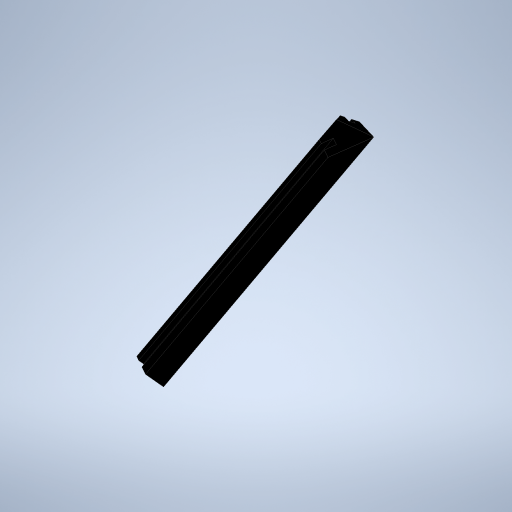
# Autodesk Inventor part: Perfil_V2
Saved by Autodesk Inventor 2024 (Build 280153000, 153)
## iProperties
Created: 2023-07-27
Part Number: Perfil_V2
Material: Genérico
Document SubType Name: Modeling
Designer: sergi
Density: 1 g/cm^3
Appearance: Valor por defecto
Author: sergi
Autodesk Inventor part; units mm, degrees
sketch "Boceto1" plane through (0, 0, 0) normal (0, 1, 0) x (-1, 0, 0)
  line L0 (65, 89.4648) -> (105.1722, -34.1725)
  line L1 (105.1722, -34.1725) -> (0, -110.5846)
  line L2 (0, -110.5846) -> (-105.1722, -34.1725)
  line L3 (-105.1722, -34.1725) -> (-65, 89.4648)
  line L4 (-65, 89.4648) -> (65, 89.4648)
  line L5 (0, 0) -> (178.9296, 0) construction
  line L6 (178.9296, 0) -> (178.9296, 178.9296) construction
  line L7 (178.9296, 178.9296) -> (0, 178.9296) construction
  line L8 (0, 178.9296) -> (0, 0) construction
  line L9 (178.9296, 178.9296) -> (0, 89.4648)
  dimension "d1" = 289.5143
  dimension "d2" = 26.565
  dimension "d108" = 130
  constraints: 20 end point, 2 horizontal, 2 midpoint, 2 parallel, 2 perpendicular, 1 coincident, 11 other
  measures "d1" distance from line of L1.end L7
  measures "d2" angle of L4 L9
  measures "d108" distance of L3.end L0.start
extrude "Extrusión1" add sketch "Boceto1" along normal blind 289.5143 draft 26.565
sketch "Boceto2" plane through (0, 289.5143, 0) normal (0, 1, 0) x (1, 0, 0)
  line L0 (0, -80.8118) -> (-76.8566, -24.9722)
  line L1 (-76.8566, -24.9722) -> (-47.5, 65.3781)
  line L2 (-47.5, 65.3781) -> (47.5, 65.3781)
  line L3 (47.5, 65.3781) -> (76.8566, -24.9722)
  line L4 (76.8566, -24.9722) -> (0, -80.8118)
  point P0 (0, 0)
  point P1 (0, 0)
  dimension "L" = 95
  constraints: 10 end point, 1 coincident, 1 horizontal, 11 other
  measures "L" distance of L1.end L2.end
extrude "Extrusión2" cut sketch "Boceto2" against normal blind 289.5143 draft 26.565 keep common part
sketch "Boceto3" plane through (65, 0, 89.4648) normal (0.8506508, -0.4472136, 0.2763932) x (0.309017, 0, -0.9510565)
  line L0 (65, 170.2767) -> (162.346, 99.5507) projected
  line L1 (-32.346, 99.5507) -> (65, 170.2767) projected
  line L2 (0, 0) -> (-32.346, 99.5507) projected
  line L3 (0, 0) -> (130, 0) projected
  line L4 (130, 0) -> (162.346, 99.5507) projected
  line L5 (151.1781, 95.922) -> (65, 158.534)
  line L6 (65, 158.534) -> (-21.1781, 95.922)
  line L7 (-21.1781, 95.922) -> (6.9022, 9.5)
  line L8 (6.9022, 9.5) -> (123.0978, 9.5)
  line L9 (123.0978, 9.5) -> (151.1781, 95.922)
  point P0 (65, -40.0099)
  dimension "D" = 9.5
  constraints: 10 end point, 4 other
  measures "D" distance between parallel lines of L4 L9
extrude "Extrusión3" cut sketch "Boceto3" against normal blind 189.5143 contours L9 L8 L7 L6 L5
sketch "Boceto4" plane through (105.1722, 0, -34.1725) normal (0.5257311, -0.4472136, -0.7236068) x (-0.809017, 0, -0.5877853)
  line L0 (65, 170.2767) -> (162.346, 99.5507) projected
  line L1 (-32.346, 99.5507) -> (65, 170.2767) projected
  line L2 (0, 0) -> (-32.346, 99.5507) projected
  line L3 (0, 0) -> (130, 0) projected
  line L4 (130, 0) -> (162.346, 99.5507) projected
  line L5 (123.0978, 9.5) -> (6.9022, 9.5)
  line L6 (6.9022, 9.5) -> (-21.1781, 95.922)
  line L7 (-21.1781, 95.922) -> (65, 158.534)
  line L8 (65, 158.534) -> (151.1781, 95.922)
  line L9 (151.1781, 95.922) -> (123.0978, 9.5)
  point P0 (65, -40.0099)
  dimension "d14" = 9.5
  constraints: 10 end point, 4 other
  measures "d14" distance between parallel lines of L3 L5
extrude "Extrusión4" cut sketch "Boceto4" against normal blind 189.5143 contours L5 L6 L7 L8 L9
sketch "Boceto5" plane through (0, 0, 0) normal (0, -1, 0) x (1, 0, 0)
  line L0 (105.1722, -34.1725) -> (0, -110.5846) projected
  line L1 (65, 89.4648) -> (105.1722, -34.1725) projected
  line L2 (-65, 89.4648) -> (65, 89.4648) projected
  line L3 (-105.1722, -34.1725) -> (-65, 89.4648) projected
  line L4 (0, -110.5846) -> (-105.1722, -34.1725) projected
  line L5 (58.0978, 79.9648) -> (94.0043, -30.5438)
  line L6 (94.0043, -30.5438) -> (0, -98.842)
  line L7 (0, -98.842) -> (-94.0043, -30.5438)
  line L8 (-94.0043, -30.5438) -> (-58.0978, 79.9648)
  line L9 (-58.0978, 79.9648) -> (58.0978, 79.9648)
  point P0 (0, 0)
  dimension "d17" = 9.5
  constraints: 10 end point, 4 other
  measures "d17" distance between parallel lines of L2 L9
extrude "Extrusión5" cut sketch "Boceto5" against normal blind 189.5143 contours L5 L6 L7 L8 L9
sketch "Boceto6" plane through (47.5, 289.5143, -65.3781) normal (0, 0.4472136, -0.8944272) x (-1, 0, 0)
  line L0 (47.5, -224.1361) -> (144.846, -153.4101) projected
  line L1 (95, 0) -> (144.846, -153.4101) projected
  line L2 (95, 0) -> (0, 0) projected
  line L3 (0, 0) -> (-49.846, -153.4101) projected
  line L4 (-49.846, -153.4101) -> (47.5, -224.1361) projected
  line L5 (133.6781, -149.7814) -> (47.5, -212.3935)
  line L6 (47.5, -212.3935) -> (-38.6781, -149.7814)
  line L7 (-38.6781, -149.7814) -> (6.9022, -9.5)
  line L8 (6.9022, -9.5) -> (88.0978, -9.5)
  line L9 (88.0978, -9.5) -> (133.6781, -149.7814)
  point P0 (47.5, -229.7114)
  dimension "d20" = 9.5
  constraints: 10 end point, 4 other
  measures "d20" distance between parallel lines of L0 L5
extrude "Extrusión6" cut sketch "Boceto6" against normal blind 189.5143 contours L5 L6 L7 L8 L9
sketch "Boceto7" plane through (0, 0, -110.5846) normal (-0.5257311, -0.4472136, -0.7236068) x (-0.809017, 0, 0.5877853)
  line L0 (65, 170.2767) -> (162.346, 99.5507) projected
  line L1 (-32.346, 99.5507) -> (65, 170.2767) projected
  line L2 (0, 0) -> (-32.346, 99.5507) projected
  line L3 (0, 0) -> (130, 0) projected
  line L4 (130, 0) -> (162.346, 99.5507) projected
  line L5 (151.1781, 95.922) -> (65, 158.534)
  line L6 (65, 158.534) -> (-21.1781, 95.922)
  line L7 (-21.1781, 95.922) -> (6.9022, 9.5)
  line L8 (6.9022, 9.5) -> (123.0978, 9.5)
  line L9 (123.0978, 9.5) -> (151.1781, 95.922)
  point P0 (65, -40.0099)
  dimension "d23" = 9.5
  constraints: 10 end point, 4 other
  measures "d23" distance between parallel lines of L4 L9
extrude "Extrusión7" cut sketch "Boceto7" against normal blind 189.5143 contours L9 L8 L7 L6 L5
sketch "Boceto8" plane through (76.8566, 289.5143, 24.9722) normal (0.8506508, 0.4472136, -0.2763932) x (-0.309017, 0, -0.9510565)
  line L0 (47.5, -224.1361) -> (144.846, -153.4101) projected
  line L1 (95, 0) -> (144.846, -153.4101) projected
  line L2 (95, 0) -> (0, 0) projected
  line L3 (0, 0) -> (-49.846, -153.4101) projected
  line L4 (-49.846, -153.4101) -> (47.5, -224.1361) projected
  line L5 (47.5, -212.3935) -> (133.6781, -149.7814)
  line L6 (133.6781, -149.7814) -> (88.0978, -9.5)
  line L7 (88.0978, -9.5) -> (6.9022, -9.5)
  line L8 (6.9022, -9.5) -> (-38.6781, -149.7814)
  line L9 (-38.6781, -149.7814) -> (47.5, -212.3935)
  point P0 (47.5, -229.7114)
  dimension "d26" = 9.5
  constraints: 10 end point, 4 other
  measures "d26" distance between parallel lines of L4 L9
extrude "Extrusión8" cut sketch "Boceto8" against normal blind 189.5143 contours L9 L8 L7 L6 L5
sketch "Boceto9" plane through (0, 289.5143, 0) normal (0, 1, 0) x (1, 0, 0)
  line L0 (78.7643, -17.095) -> (-82.4461, -69.4755) projected
  line L1 (-47.5, 65.3781) -> (47.5, 65.3781) projected
  line L2 (-76.8566, -24.9722) -> (-47.5, 65.3781) projected
  line L3 (0, -80.8118) -> (-76.8566, -24.9722) projected
  line L4 (76.8566, -24.9722) -> (0, -80.8118) projected
  line L5 (47.5, 65.3781) -> (76.8566, -24.9722) projected
  line L6 (0, -69.0692) -> (-65.6887, -21.3436)
  line L7 (-65.6887, -21.3436) -> (-40.5978, 55.8781)
  line L8 (-40.5978, 55.8781) -> (40.5978, 55.8781)
  line L9 (40.5978, 55.8781) -> (65.6887, -21.3436)
  line L10 (65.6887, -21.3436) -> (0, -69.0692)
  point P0 (0, 0)
  dimension "d29" = 9.5
  constraints: 10 end point, 4 other
  measures "d29" distance between parallel lines of L4 L10
extrude "Extrusión9" cut sketch "Boceto9" against normal blind 189.5143 contours L10 L6 L0 | L0 L6 L7 L8 L9
sketch "Boceto10" plane through (-47.5, 289.5143, -65.3781) normal (-0.8506508, 0.4472136, -0.2763932) x (-0.309017, 0, 0.9510565)
  line L0 (-49.846, -153.4101) -> (47.5, -224.1361) projected
  line L1 (47.5, -224.1361) -> (144.846, -153.4101) projected
  line L2 (95, 0) -> (144.846, -153.4101) projected
  line L3 (95, 0) -> (0, 0) projected
  line L4 (0, 0) -> (-49.846, -153.4101) projected
  line L5 (133.6781, -149.7814) -> (47.5, -212.3935)
  line L6 (47.5, -212.3935) -> (-38.6781, -149.7814)
  line L7 (-38.6781, -149.7814) -> (6.9022, -9.5)
  line L8 (6.9022, -9.5) -> (88.0978, -9.5)
  line L9 (88.0978, -9.5) -> (133.6781, -149.7814)
  point P0 (47.5, -229.7114)
  dimension "d32" = 9.5
  constraints: 10 end point, 4 other
  measures "d32" distance between parallel lines of L2 L9
extrude "Extrusión10" cut sketch "Boceto10" against normal blind 189.5143 contours L5 L6 L7 L8 L9
sketch "Boceto11" plane through (-105.1722, 0, -34.1725) normal (-0.8506508, -0.4472136, 0.2763932) x (0.309017, 0, 0.9510565)
  line L0 (93.5693, 85.4327) -> (113.4241, 91.884) projected
  line L1 (-32.346, 99.5507) -> (65, 170.2767) projected
  line L2 (0, 0) -> (-32.346, 99.5507) projected
  line L3 (0, 0) -> (130, 0) projected
  line L4 (130, 0) -> (162.346, 99.5507) projected
  line L5 (65, 170.2767) -> (162.346, 99.5507) projected
  line L6 (151.1781, 95.922) -> (123.0978, 9.5)
  line L7 (123.0978, 9.5) -> (6.9022, 9.5)
  line L8 (6.9022, 9.5) -> (-21.1781, 95.922)
  line L9 (-21.1781, 95.922) -> (65, 158.534)
  line L10 (65, 158.534) -> (151.1781, 95.922)
  point P0 (65, -40.0099)
  point P1 (48.882, 67.2803)
  point P2 (90.6407, 79.3954)
  point P3 (78.7461, 79.1633)
  dimension "d35" = 9.5
  constraints: 10 end point, 5 other
  measures "d35" distance between parallel lines of L4 L6
extrude "Extrusión11" cut sketch "Boceto11" against normal blind 189.5143 contours L6 L7 L8 L9 L10
sketch "Boceto12" plane through (-65, 0, 89.4648) normal (0, -0.4472136, 0.8944272) x (1, 0, 0)
  line L0 (6.9022, 9.5) -> (97.7716, 134.5711) projected
  line L1 (-32.346, 99.5507) -> (65, 170.2767) projected
  line L2 (0, 0) -> (-32.346, 99.5507) projected
  line L3 (0, 0) -> (130, 0) projected
  line L4 (130, 0) -> (162.346, 99.5507) projected
  line L5 (65, 170.2767) -> (162.346, 99.5507) projected
  line L6 (151.1781, 95.922) -> (123.0978, 9.5)
  line L7 (123.0978, 9.5) -> (6.9022, 9.5)
  line L8 (6.9022, 9.5) -> (-21.1781, 95.922)
  line L9 (-21.1781, 95.922) -> (65, 158.534)
  line L10 (65, 158.534) -> (151.1781, 95.922)
  point P0 (65, -40.0099)
  point P1 (52.5, 72.2601)
  point P2 (45.5555, 62.7017)
  dimension "d38" = 9.5
  constraints: 10 end point, 4 other
  measures "d38" distance between parallel lines of L5 L10
extrude "Extrusión12" cut sketch "Boceto12" against normal blind 189.5143 contours L6 L7 L8 L9 L10
sketch "Boceto13" plane through (0, 289.5143, 80.8118) normal (0.5257311, 0.4472136, 0.7236068) x (0.809017, 0, -0.5877853)
  line L0 (-49.846, -153.4101) -> (47.5, -224.1361) projected
  line L1 (47.5, -224.1361) -> (144.846, -153.4101) projected
  line L2 (95, 0) -> (144.846, -153.4101) projected
  line L3 (95, 0) -> (0, 0) projected
  line L4 (0, 0) -> (-49.846, -153.4101) projected
  line L5 (47.5, -212.3935) -> (-38.6781, -149.7814)
  line L6 (-38.6781, -149.7814) -> (6.9022, -9.5)
  line L7 (6.9022, -9.5) -> (88.0978, -9.5)
  line L8 (88.0978, -9.5) -> (133.6781, -149.7814)
  line L9 (133.6781, -149.7814) -> (47.5, -212.3935)
  point P0 (47.5, -229.7114)
  dimension "d41" = 9.5
  constraints: 10 end point, 4 other
  measures "d41" distance between parallel lines of L0 L5
extrude "Extrusión13" cut sketch "Boceto13" against normal blind 189.5143 contours L5 L6 L7 L8 L9
sketch "Boceto14" plane through (-76.8566, 289.5143, 24.9722) normal (-0.5257311, 0.4472136, 0.7236068) x (0.809017, 0, 0.5877853)
  line L0 (-49.846, -153.4101) -> (47.5, -224.1361) projected
  line L1 (47.5, -224.1361) -> (144.846, -153.4101) projected
  line L2 (95, 0) -> (144.846, -153.4101) projected
  line L3 (95, 0) -> (0, 0) projected
  line L4 (0, 0) -> (-49.846, -153.4101) projected
  line L5 (-38.6781, -149.7814) -> (47.5, -212.3935)
  line L6 (47.5, -212.3935) -> (133.6781, -149.7814)
  line L7 (133.6781, -149.7814) -> (88.0978, -9.5)
  line L8 (88.0978, -9.5) -> (6.9022, -9.5)
  line L9 (6.9022, -9.5) -> (-38.6781, -149.7814)
  point P0 (47.5, -229.7114)
  dimension "d44" = 9.5
  constraints: 10 end point, 4 other
  measures "d44" distance between parallel lines of L4 L9
extrude "Extrusión14" cut sketch "Boceto14" against normal blind 189.5143 contours L9 L8 L7 L6 L5
ref_plane "Plano de trabajo1" through (47.5, 288.1726, -62.6949) normal (0, 0.4472136, -0.8944272) x (-1, 0, 0)
sketch "Boceto15" plane through (47.5, 288.1726, -62.6949) normal (0, 0.4472136, -0.8944272) x (-1, 0, 0)
  line L0 (6.9022, -9.5) -> (88.0978, -9.5) projected
  line L1 (-38.6781, -149.7814) -> (6.9022, -9.5) projected
  line L2 (47.5, -212.3935) -> (-38.6781, -149.7814) projected
  line L3 (133.6781, -149.7814) -> (47.5, -212.3935) projected
  line L4 (88.0978, -9.5) -> (133.6781, -149.7814) projected
  line L5 (5.0858, -7) -> (89.9142, -7)
  line L6 (89.9142, -7) -> (136.617, -150.7364)
  line L7 (136.617, -150.7364) -> (47.5, -215.4836)
  line L8 (47.5, -215.4836) -> (-41.617, -150.7364)
  line L9 (-41.617, -150.7364) -> (5.0858, -7)
  point P0 (47.5, -229.7114)
  dimension "D2" = 2.5
  constraints: 10 end point, 4 other
  measures "D2" distance between parallel lines of L1 L9
extrude "Extrusión15" cut sketch "Boceto15" along normal mid plane 1.8 contours L0 L4 L3 L2 L1 | L5 L6 L7 L8 L9
ref_plane "Plano de trabajo2" through (103.595, 1.3416, -32.0017) normal (0.5257311, -0.4472136, -0.7236068) x (-0.809017, 0, -0.5877853)
sketch "Boceto16" plane through (103.595, 1.3416, -32.0017) normal (0.5257311, -0.4472136, -0.7236068) x (-0.809017, 0, -0.5877853)
  line L0 (123.0978, 9.5) -> (6.9022, 9.5) projected
  line L1 (151.1781, 95.922) -> (123.0978, 9.5) projected
  line L2 (65, 158.534) -> (151.1781, 95.922) projected
  line L3 (-21.1781, 95.922) -> (65, 158.534) projected
  line L4 (6.9022, 9.5) -> (-21.1781, 95.922) projected
  line L5 (5.0858, 7) -> (124.9142, 7)
  line L6 (124.9142, 7) -> (154.117, 96.8769)
  line L7 (154.117, 96.8769) -> (65, 161.6242)
  line L8 (65, 161.6242) -> (-24.117, 96.8769)
  line L9 (-24.117, 96.8769) -> (5.0858, 7)
  point P0 (65, -40.0099)
  dimension "d52" = 2.5
  constraints: 10 end point, 4 other
  measures "d52" distance between parallel lines of L0 L5
extrude "Extrusión16" cut sketch "Boceto16" along normal mid plane 1.8
ref_plane "Plano de trabajo3" through (74.3047, 288.1726, 25.8014) normal (0.8506508, 0.4472136, -0.2763932) x (-0.309017, 0, -0.9510565)
sketch "Boceto17" plane through (74.3047, 288.1726, 25.8014) normal (0.8506508, 0.4472136, -0.2763932) x (-0.309017, 0, -0.9510565)
  line L0 (47.5, -212.3935) -> (-38.6781, -149.7814) projected
  line L1 (133.6781, -149.7814) -> (47.5, -212.3935) projected
  line L2 (88.0978, -9.5) -> (133.6781, -149.7814) projected
  line L3 (6.9022, -9.5) -> (88.0978, -9.5) projected
  line L4 (-38.6781, -149.7814) -> (6.9022, -9.5) projected
  line L5 (-41.617, -150.7364) -> (47.5, -215.4836)
  line L6 (47.5, -215.4836) -> (136.617, -150.7364)
  line L7 (136.617, -150.7364) -> (89.9142, -7)
  line L8 (89.9142, -7) -> (5.0858, -7)
  line L9 (5.0858, -7) -> (-41.617, -150.7364)
  point P0 (47.5, -229.7114)
  dimension "d56" = 2.5
  constraints: 10 end point, 4 other
  measures "d56" distance between parallel lines of L0 L5
extrude "Extrusión17" cut sketch "Boceto17" along normal mid plane 1.8
ref_plane "Plano de trabajo4" through (1.5772, 1.3416, -108.4138) normal (-0.5257311, -0.4472136, -0.7236068) x (-0.809017, 0, 0.5877853)
sketch "Boceto18" plane through (1.5772, 1.3416, -108.4138) normal (-0.5257311, -0.4472136, -0.7236068) x (-0.809017, 0, 0.5877853)
  line L0 (151.1781, 95.922) -> (123.0978, 9.5) projected
  line L1 (65, 158.534) -> (151.1781, 95.922) projected
  line L2 (-21.1781, 95.922) -> (65, 158.534) projected
  line L3 (6.9022, 9.5) -> (-21.1781, 95.922) projected
  line L4 (123.0978, 9.5) -> (6.9022, 9.5) projected
  line L5 (124.9142, 7) -> (154.117, 96.8769)
  line L6 (154.117, 96.8769) -> (65, 161.6242)
  line L7 (65, 161.6242) -> (-24.117, 96.8769)
  line L8 (-24.117, 96.8769) -> (5.0858, 7)
  line L9 (5.0858, 7) -> (124.9142, 7)
  point P0 (65, -40.0099)
  dimension "d60" = 2.5
  constraints: 10 end point, 4 other
  measures "d60" distance between parallel lines of L0 L5
extrude "Extrusión18" cut sketch "Boceto18" along normal mid plane 1.8 contours L0 L4 L3 L2 L1 | L9 L8 L7 L6 L5
ref_plane "Plano de trabajo5" through (0, 3, 0) normal (0, -1, 0) x (1, 0, 0)
sketch "Boceto19" plane through (0, 3, 0) normal (0, -1, 0) x (1, 0, 0)
  line L0 (0, -98.842) -> (-94.0043, -30.5438) projected
  line L1 (-94.0043, -30.5438) -> (-58.0978, 79.9648) projected
  line L2 (-58.0978, 79.9648) -> (58.0978, 79.9648) projected
  line L3 (58.0978, 79.9648) -> (94.0043, -30.5438) projected
  line L4 (94.0043, -30.5438) -> (0, -98.842) projected
  line L5 (105.1722, -34.1725) -> (0, -110.5846) projected
  line L6 (65, 89.4648) -> (105.1722, -34.1725) projected
  line L7 (-65, 89.4648) -> (65, 89.4648) projected
  line L8 (-105.1722, -34.1725) -> (-65, 89.4648) projected
  line L9 (0, -110.5846) -> (-105.1722, -34.1725) projected
  line L10 (-59.9142, 82.4648) -> (-96.9432, -31.4988)
  line L11 (-96.9432, -31.4988) -> (0, -101.9321)
  line L12 (0, -101.9321) -> (96.9432, -31.4988)
  line L13 (96.9432, -31.4988) -> (59.9142, 82.4648)
  line L14 (59.9142, 82.4648) -> (-59.9142, 82.4648)
  point P0 (0, 0)
  dimension "d64" = 2.5
  constraints: 10 end point, 4 other
  measures "d64" distance between parallel lines of L1 L10
extrude "Extrusión19" cut sketch "Boceto19" along normal mid plane 1.8 contours L0 L1 L2 L3 L4 | L14 L13 L12 L11 L10
ref_plane "Plano de trabajo6" through (62.448, 1.3416, 88.6356) normal (0.8506508, -0.4472136, 0.2763932) x (0.309017, 0, -0.9510565)
sketch "Boceto20" plane through (62.448, 1.3416, 88.6356) normal (0.8506508, -0.4472136, 0.2763932) x (0.309017, 0, -0.9510565)
  line L0 (6.9022, 9.5) -> (-21.1781, 95.922) projected
  line L1 (-21.1781, 95.922) -> (65, 158.534) projected
  line L2 (65, 158.534) -> (151.1781, 95.922) projected
  line L3 (151.1781, 95.922) -> (123.0978, 9.5) projected
  line L4 (123.0978, 9.5) -> (6.9022, 9.5) projected
  line L5 (65, 170.2767) -> (162.346, 99.5507) projected
  line L6 (-32.346, 99.5507) -> (65, 170.2767) projected
  line L7 (0, 0) -> (-32.346, 99.5507) projected
  line L8 (0, 0) -> (130, 0) projected
  line L9 (130, 0) -> (162.346, 99.5507) projected
  line L10 (-24.117, 96.8769) -> (5.0858, 7)
  line L11 (5.0858, 7) -> (124.9142, 7)
  line L12 (124.9142, 7) -> (154.117, 96.8769)
  line L13 (154.117, 96.8769) -> (65, 161.6242)
  line L14 (65, 161.6242) -> (-24.117, 96.8769)
  point P0 (65, -40.0099)
  dimension "d68" = 2.5
  constraints: 10 end point, 4 other
  measures "d68" distance between parallel lines of L0 L10
extrude "Extrusión20" cut sketch "Boceto20" along normal mid plane 1.8 contours L0 L1 L2 L3 L4 | L14 L13 L12 L11 L10
ref_plane "Plano de trabajo7" through (152.5146, 99.5438, -49.555) normal (-0.309017, 0, -0.9510565) x (-0.8506508, -0.4472136, 0.2763932)
split body "Dividir1" result two bodies by plane through (152.5146, 99.5438, -49.555) normal (-0.309017, 0, -0.9510565) first body at (-65.7478, 240.7202, -86.3585)
ref_plane "Plano de trabajo8" through (147.5202, 85.7952, -56.4293) normal (0, -0.8506508, 0.5257311) x (-0.5257311, 0.4472136, 0.7236068)
split "Dividir2" plane through (147.5202, 85.7952, -56.4293) removes the side toward (0, 0.8506508, -0.5257311)
ref_plane "Plano de trabajo9" through (152.5146, 85.7952, -41.058) normal (-0.309017, -0.8506508, -0.4253254) x (-0.8506508, 0.4472136, -0.2763932)
split "Dividir3" plane through (152.5146, 85.7952, -41.058) removes the side toward (0.309017, 0.8506508, 0.4253254)
ref_plane "Plano de trabajo13" through (47.0021, 15.3713, -64.6929) normal (-0.5, -0.5257311, 0.688191) x (0.809017, 0, 0.5877853)
split "Dividir7" plane through (47.0021, 15.3713, -64.6929) removes the side toward (-0.5, -0.5257311, 0.688191)
ref_plane "Plano de trabajo14" through (102.0855, 8.4971, -41.6666) normal (-0.809017, -0.5257311, -0.2628656) x (-0.5257311, 0.4472136, 0.7236068)
split "Dividir8" plane through (102.0855, 8.4971, -41.6666) removes the side toward (-0.809017, -0.5257311, -0.2628656)
ref_plane "Plano de trabajo16" through (137.7424, 69.9535, -38.414) normal (-0.809017, 0.5257311, 0.2628656) x (0.5, 0.8506508, -0.1624598)
ref_plane "Plano de trabajo15" through (138.5514, 69.4278, -38.6769) normal (-0.809017, 0.5257311, 0.2628656) x (0.5, 0.8506508, -0.1624598)
combine bodies "Combinar1" operation type add bodies to combine 2 3
split "Dividir9" plane through (137.7424, 69.9535, -38.414) removes the side toward (-0.809017, 0.5257311, 0.2628656)
sketch "Boceto25" plane through (99.4171, 10.7669, -37.9939) normal (-0.809017, 0.5257311, 0.2628656) x (0.309017, 0, 0.9510565)
  line L0 (5.4128, -6.9022) -> (5.4128, 97.7716) projected
  line L1 (0, 90.8695) -> (5.4128, 94.2147) projected
  line L2 (0, 0) -> (0, 90.8695) projected
  line L3 (5.4128, -3.3453) -> (0, 0) projected
  line L4 (10.8256, 0) -> (5.4128, -3.3453) projected
  line L5 (10.8256, 90.8695) -> (10.8256, 0) projected
  line L6 (5.4128, 94.2147) -> (10.8256, 90.8695) projected
  point P0 (5.4128, -65.0399)
  dimension "d109" = 10.8256
  measures "d109" distance between parallel lines of L5 L2
equation "\"d3\" = d1"
equation "\"d4\" = d2"
equation "\"d6\" = d1"
equation "\"d7\" = d2"
equation "\"d14\" = D"
equation "\"d17\" = D"
equation "\"d20\" = D"
equation "\"d23\" = D"
equation "\"d26\" = D"
equation "\"d29\" = D"
equation "\"d32\" = D"
equation "\"d35\" = D"
equation "\"d38\" = D"
equation "\"d41\" = D"
equation "\"d44\" = D"
equation "\"d48\" = ESP"
equation "\"d52\" = D2"
equation "\"d56\" = D2"
equation "\"d57\" = ESP"
equation "\"d60\" = D2"
equation "\"d61\" = ESP"
equation "\"d64\" = D2"
equation "\"d65\" = ESP"
equation "\"d68\" = D2"
equation "\"d69\" = ESP"
equation "\"d51\" = P"
equation "\"d55\" = P"
equation "\"d59\" = P"
equation "\"d63\" = P"
equation "\"d67\" = P"
equation "\"ESP\" = 1.8"
equation "\"P\" = -3"
